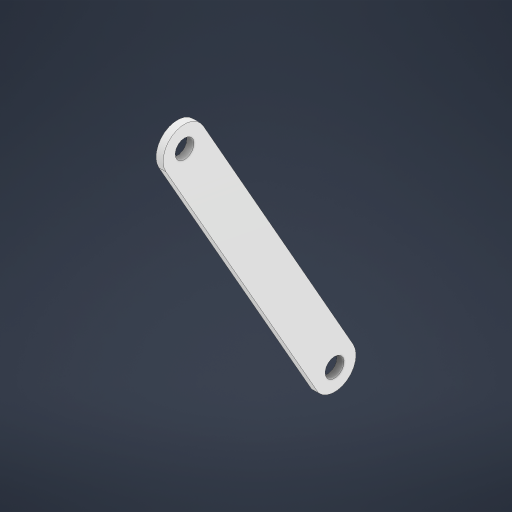
# Autodesk Inventor part: battery_mount_arm
Saved by Autodesk Inventor 2024 (Build 280153000, 153)
## iProperties
Created: 2023-11-22
Part Number: battery_mount_arm
Material: Acetal Resin, White
Document SubType Name: Modeling
Designer: avere
Density: 1.425 g/cm^3
Appearance: Smooth - White
Author: avere
Autodesk Inventor part; units mm, degrees
ref_plane "YZ Plane" through (0, 0, 0) normal (1, 0, 0) x (0, 1, 0)
ref_plane "XZ Plane" through (0, 0, 0) normal (0, 1, 0) x (-1, 0, 0)
ref_plane "XY Plane" through (0, 0, 0) normal (0, 0, 1) x (1, 0, 0)
sketch "Sketch1" plane through (0, 0, 0) normal (1, 0, 0) x (0, 1, 0)
  circle A0 centre (-29.1044, -27.1833) radius 2.1082
  arc A1 (-30.5385, -22.6419) -> (-26.7536, -31.3252) centre (-29.1044, -27.1833) ccw
  circle A2 centre (29.6331, 6.1542) radius 2.0955
  arc A3 (31.9839, 2.0123) -> (27.2758, 10.2924) centre (29.6331, 6.1542) ccw
  line L0 (-32.2794, -23.6335) -> (27.2758, 10.2924)
  line L1 (31.9839, 2.0123) -> (-26.7536, -31.3252)
  point P0 (0, 0)
  dimension "d0" = 9.525
  dimension "d1" = 9.525
  constraints: 6 point on circle, 4 centre point, 4 end point, 2 coincident, 2 point on line, 2 tangent, 2 other
  measures "d0" diameter of A1
  measures "d1" diameter of A3
extrude "Extrusion1" add sketch "Sketch1" along normal blind 1.5875 contours L0 A3 L1 A1
body "Solid1"
